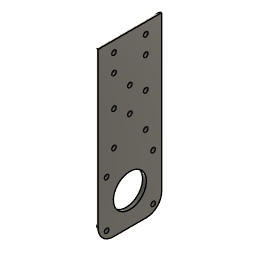
CHASSI_SideFrame_RIGHT (Autodesk Fusion 360 design; units mm, degrees)
Autodesk Fusion 360 part; units mm, degrees
sketch "Sketch1" plane through (0, 0, 0) normal (1, 0, 0) x (0, 1, 0)
  line L0 (-21.15, 21.15) -> (-21.15, -11.15)
  line L1 (-11.15, -21.15) -> (11.15, -21.15)
  line L2 (21.15, -11.15) -> (21.15, -6)
  line L3 (0, 21.15) -> (0, -21.15) construction
  circle A0 centre (15.5, 15.5) radius 1.5
  circle A1 centre (-15.5, 15.5) radius 1.5
  line L4 (21.15, 0) -> (-21.15, 0) construction
  circle A2 centre (-15.5, -15.5) radius 1.5
  circle A3 centre (15.5, -15.5) radius 1.5
  circle A4 centre (0, 0) radius 11
  arc A5 (11.15, -21.15) -> (21.15, -11.15) centre (11.15, -11.15) ccw
  arc A6 (-21.15, -11.15) -> (-11.15, -21.15) centre (-11.15, -11.15) ccw
  line L5 (21.15, -6) -> (-21.15, -6) construction
  line L6 (-21.15, -6) -> (-21.15, 92)
  line L7 (-21.15, 92) -> (21.15, 92)
  line L8 (21.15, 92) -> (21.15, -6)
  point P0 (-21.15, -21.15)
  point P1 (21.15, -21.15)
  dimension "d1_1" = 42.3
  dimension "d2_1" = 42.3
  dimension "d3_1" = 3
  dimension "d4_1" = 3
  dimension "d5_1" = 15.5
  dimension "d6_1" = 15.5
  dimension "d7_1" = 15.5
  dimension "d8_1" = 15.5
  dimension "d9_1" = 22
  dimension "d10_1" = 10
  dimension "d11_1" = 98
  constraint parallel L0 L2
  constraint coincident A4.centre origin
  constraint symmetric A0 L4 A3
  constraint symmetric A1 L4 A2
  constraint coincident L1 L3.end
  constraint coincident L2 L4.start
  constraint coincident P1 L1
  constraint coincident P1 L2
  constraint tangent L1 A5
  constraint tangent L2 A5
  constraint coincident L0 L4.end
  constraint coincident P0 L0
  constraint coincident P0 L1
  constraint tangent L0 A6
  constraint tangent L1 A6
  constraint equal A5 A6
  constraint horizontal L5
  constraint vertical L6
  constraint horizontal L7
  constraint vertical L8
  measures "d1_1" distance of P0 P1
  measures "d2_1" distance of L0.start P0
  measures "d3_1" diameter of A0
  measures "d4_1" diameter of A1
  measures "d5_1" distance of L3 A1.centre
  measures "d6_1" distance of A1.centre L4
  measures "d7_1" distance of A0.centre L4
  measures "d8_1" distance of L3 A0.centre
  measures "d9_1" diameter of A4
  measures "d10_1" radius of A5
  measures "d11_1" distance of L2.end L7.end
extrude "Extrude1" add sketch "Sketch1" along normal blind 2.5
sketch "Sketch2" plane through (0, 0, 0) normal (-1, 0, 0) x (0, -1, 0)
  circle A0 centre (15.5, -15.5) radius 1.5
  circle A1 centre (15.5, 15.5) radius 1.5
  circle A2 centre (0, 0) radius 11
  circle A3 centre (-15.5, -15.5) radius 1.5
  circle A4 centre (-15.5, 15.5) radius 1.5
  line L0 (21.15, -11.15) -> (21.15, 92)
  line L1 (21.15, 92) -> (-21.15, 92)
  line L2 (-21.15, 92) -> (-21.15, -11.15)
  arc A5 (-21.15, -11.15) -> (-11.15, -21.15) centre (-11.15, -11.15) ccw
  line L3 (-11.15, -21.15) -> (11.15, -21.15)
  arc A6 (11.15, -21.15) -> (21.15, -11.15) centre (11.15, -11.15) ccw
  circle A7 centre (0, 60.75) radius 1.5
  circle A8 centre (10.575, 52.5) radius 1.5
  circle A9 centre (-10.575, 52.5) radius 1.5
  circle A10 centre (0, 44.25) radius 1.5
  line L4 (21.15, 36) -> (21.15, 69)
  line L5 (21.15, 69) -> (-21.15, 69)
  line L6 (-21.15, 69) -> (-21.15, 36)
  line L7 (-21.15, 36) -> (21.15, 36)
  circle A11 centre (-10.575, 52.5) radius 1.5
  circle A12 centre (0, 60.75) radius 1.5
  circle A13 centre (10.575, 52.5) radius 1.5
  circle A14 centre (0, 44.25) radius 1.5
  dimension "d29" = 3
  dimension "d30" = 3
  dimension "d31" = 3
  dimension "d32" = 3
  constraint concentric A9 A11
  constraint concentric A7 A12
  constraint concentric A8 A13
  constraint concentric A10 A14
  measures "d29" diameter of A11
  measures "d30" diameter of A12
  measures "d31" diameter of A13
  measures "d32" diameter of A14
extrude "Extrude2" cut sketch "Sketch2" against normal blind 2.5 contours A7 A12 | A8 A13 | A9 A11 | A10 A14
sketch "Sketch3" plane through (0, 0, 0) normal (-1, 0, 0) x (0, -1, 0)
  circle A0 centre (0, 60.75) radius 1.5
  circle A1 centre (10.575, 52.5) radius 1.5
  circle A2 centre (-10.575, 52.5) radius 1.5
  circle A3 centre (0, 44.25) radius 1.5
  circle A4 centre (-15.5, -15.5) radius 1.5
  circle A5 centre (15.5, -15.5) radius 1.5
  circle A6 centre (15.5, 15.5) radius 1.5
  circle A7 centre (0, 0) radius 11
  circle A8 centre (-15.5, 15.5) radius 1.5
  line L0 (21.15, -11.15) -> (21.15, 92)
  line L1 (21.15, 92) -> (-21.15, 92)
  line L2 (-21.15, 92) -> (-21.15, -11.15)
  arc A9 (-21.15, -11.15) -> (-11.15, -21.15) centre (-11.15, -11.15) ccw
  line L3 (-11.15, -21.15) -> (11.15, -21.15)
  arc A10 (11.15, -21.15) -> (21.15, -11.15) centre (11.15, -11.15) ccw
  circle A11 centre (10.575, 84.8108) radius 1.5
  circle A12 centre (-10.575, 84.8108) radius 1.5
  circle A13 centre (0, 60.75) radius 1.5
  circle A14 centre (-10.575, 52.5) radius 1.5
  circle A15 centre (10.575, 52.5) radius 1.5
  circle A16 centre (0, 44.25) radius 1.5
  circle A17 centre (15.5, 15.5) radius 1.5
  circle A18 centre (-15.5, 15.5) radius 1.5
  circle A19 centre (-15.5, -15.5) radius 1.5
  circle A20 centre (15.5, -15.5) radius 1.5
  circle A21 centre (0, 0) radius 11
  line L4 (21.15, 92) -> (21.15, -11.15)
  arc A22 (11.15, -21.15) -> (21.15, -11.15) centre (11.15, -11.15) ccw
  line L5 (11.15, -21.15) -> (-11.15, -21.15)
  arc A23 (-21.15, -11.15) -> (-11.15, -21.15) centre (-11.15, -11.15) ccw
  line L6 (-21.15, -11.15) -> (-21.15, 92)
  line L7 (-21.15, 92) -> (21.15, 92)
extrude "Extrude3" cut sketch "Sketch3" against normal blind 2.5 contours A11 | A12
fillet "Fillet1" radius 2.5 6 edges at (0, 0, 92) (0, 21.15, 40.425) (0, 18.2211, -18.2211) (0, 0, -21.15) (0, -18.2211, -18.2211) (0, -21.15, 40.425)
sketch "Sketch4" plane through (0, 0, 0) normal (-1, 0, 0) x (0, -1, 0)
  circle A0 centre (-15.5, 15.5) radius 1.5
  circle A1 centre (0, 0) radius 11
  circle A2 centre (15.5, 15.5) radius 1.5
  arc A3 (16.9413, -15.9156) -> (18.65, -11.15) centre (11.15, -11.15) ccw
  line L0 (18.65, -11.15) -> (18.65, 89.5)
  line L1 (18.65, 89.5) -> (-18.65, 89.5)
  line L2 (-18.65, 89.5) -> (-18.65, -11.15)
  arc A4 (-18.65, -11.15) -> (-16.9413, -15.9156) centre (-11.15, -11.15) ccw
  arc A5 (-15.9156, -16.9413) -> (-16.9413, -15.9156) centre (-15.5, -15.5) ccw
  arc A6 (-15.9156, -16.9413) -> (-11.15, -18.65) centre (-11.15, -11.15) ccw
  line L3 (-11.15, -18.65) -> (11.15, -18.65)
  arc A7 (11.15, -18.65) -> (15.9156, -16.9413) centre (11.15, -11.15) ccw
  arc A8 (16.9413, -15.9156) -> (15.9156, -16.9413) centre (15.5, -15.5) ccw
  circle A9 centre (0, 44.25) radius 1.5
  circle A10 centre (-10.575, 52.5) radius 1.5
  circle A11 centre (10.575, 52.5) radius 1.5
  circle A12 centre (0, 60.75) radius 1.5
  circle A13 centre (10.575, 84.8108) radius 1.5
  circle A14 centre (-10.575, 84.8108) radius 1.5
  line L4 (0, 15.5) -> (0, 44.25) construction
  line L5 (-18.65, 29.8573) -> (18.65, 29.8573) construction
  line L6 (-10.575, 52.5) -> (-10.575, 29.8573) construction
  line L7 (10.575, 52.5) -> (10.575, 29.8573) construction
  circle A15 centre (-10.575, 29.8573) radius 1.5
  circle A16 centre (10.575, 29.8573) radius 1.5
  line L8 (0, 60.75) -> (0, 84.8108) construction
  line L9 (-18.65, 73.0231) -> (18.65, 73.0231) construction
  line L10 (-10.575, 52.5) -> (-10.575, 73.0231) construction
  line L11 (10.575, 52.5) -> (10.575, 73.0231) construction
  circle A17 centre (-10.575, 73.0231) radius 1.5
  circle A18 centre (10.575, 73.0231) radius 1.5
  dimension "d360" = 3
  dimension "d361" = 3
  dimension "d362" = 3
  dimension "d363" = 3
  constraint coincident A9.centre L4.end
  constraint vertical L4
  constraint coincident L2 L5.start
  constraint coincident L0 L5.end
  constraint perpendicular L0 L5
  constraint coincident A10.centre L6.start
  constraint coincident L5 L6.end
  constraint perpendicular L5 L6
  constraint coincident A11.centre L7.start
  constraint coincident L5 L7.end
  constraint perpendicular L5 L7
  constraint coincident L6.end A15.centre
  constraint coincident L7.end A16.centre
  constraint coincident A12.centre L8.start
  constraint perpendicular L1 L8
  constraint coincident L2 L9.start
  constraint coincident L0 L9.end
  constraint perpendicular L0 L9
  constraint perpendicular L9 L10
  constraint coincident L9 L11.end
  constraint perpendicular L9 L11
  constraint coincident L10.end A17.centre
  constraint coincident L11.end A18.centre
  measures "d360" diameter of A15
  measures "d361" diameter of A16
  measures "d362" diameter of A17
  measures "d363" diameter of A18
extrude "Extrude4" cut sketch "Sketch4" against normal blind 2.5 contours A15 | A16 | A17 | A18
